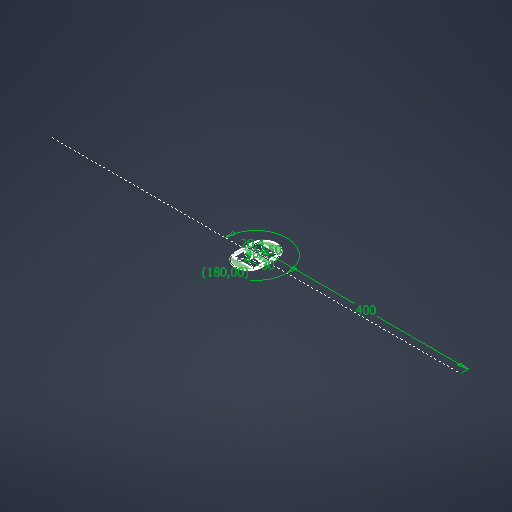
# Autodesk Inventor part: base
Saved by Autodesk Inventor 2027 (Build 310192060, 192F)
## iProperties
Created: 2026-08-01
Part Number: base
Material: Ogólny
Document SubType Name: Modeling
Designer: User
Density: 1 g/cm^3
Appearance: Domyślna
Author: User
Autodesk Inventor part; units mm, degrees
ref_plane "YZ Plane" through (0, 0, 0) normal (1, 0, 0) x (0, 1, 0)
ref_plane "XZ Plane" through (0, 0, 0) normal (0, 1, 0) x (-1, 0, 0)
ref_plane "XY Plane" through (0, 0, 0) normal (0, 0, 1) x (1, 0, 0)
sketch "Szkic1" plane through (0, 0, 0) normal (0, 1, 0) x (-1, 0, 0)
  line L0 (0, 0) -> (0, -30)
  circle A0 centre (0, 0) radius 2
  circle A1 centre (0, -30) radius 2
  line L1 (0, 0) -> (0, -30) construction
  line L2 (-25, 0) -> (-25, -30)
  line L3 (25, -30) -> (25, 0)
  arc A2 (25, 0) -> (-25, 0) centre (0, 0) ccw
  arc A3 (-25, -30) -> (25, -30) centre (0, -30) ccw
  line L4 (-20.2, -40.2) -> (20.2, -40.2)
  line L5 (20.2, -40.2) -> (20.2, -19.8)
  line L6 (20.2, -19.8) -> (-20.2, -19.8)
  line L7 (-20.2, -19.8) -> (-20.2, -40.2)
  line L8 (-20.2, -40.2) -> (20.2, -19.8) construction
  line L9 (20.2, -40.2) -> (-20.2, -19.8) construction
  line L10 (0, -15) -> (-25, -15) construction
  line L11 (0, -30) -> (0, 0)
  circle A4 centre (0, 0) radius 2
  line L12 (0, -30) -> (0, 0) construction
  line L13 (-20.2, 10.2) -> (20.2, 10.2)
  line L14 (20.2, 10.2) -> (20.2, -10.2)
  line L15 (20.2, -10.2) -> (-20.2, -10.2)
  line L16 (-20.2, 10.2) -> (20.2, -10.2) construction
  line L17 (20.2, 10.2) -> (-20.2, -10.2) construction
  line L18 (-20.2, -10.2) -> (-20.2, 10.2)
  line L19 (0, -15) -> (-400, -15) construction
  line L20 (0, -15) -> (400, -15) construction
  dimension "d0" = 30
  dimension "d1" = 4
  dimension "d2" = 4
  dimension "d3" = 50
  dimension "d6" = 40.4
  dimension "d7" = 20.4
  dimension "d8" = 400
  dimension "d9" = 180
  constraints: 46 end point, 8 symmetric about line, 5 centre point, 4 coincident, 4 midpoint, 4 point on circle, 4 tangent, 3 collinear, 3 parallel, 2 horizontal, 2 vertical, 1 perpendicular, 1 other
  measures "d0" distance of L0.start L0.end
  measures "d1" diameter of A0
  measures "d2" diameter of A1
  measures "d3" diameter of A3
  measures "d6" distance of L6.end L5.end
  measures "d7" distance of L5.end L4.end
  measures "d8" distance of L10.start L19.end
  measures "d9" angle of L20 L19
extrude "Wyciągnięcie proste1" add sketch "Szkic1" against normal blind 2 contours A2 L3 A3 L2
